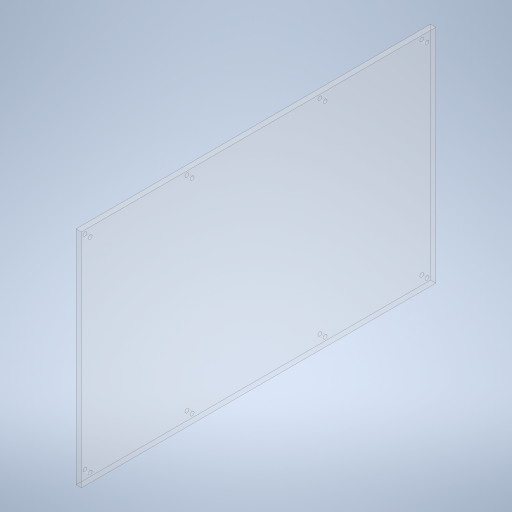
# Autodesk Inventor part: Perspex_plaat
Saved by Autodesk Inventor 2023 (Build 270158000, 158)
## iProperties
Created: 2022-09-12
Part Number: Perspex_plaat
Material: Polycarbonate, Clear
Document SubType Name: Modeling
Designer: VoorL
Density: 1.2 g/cm^3
Appearance: Polycarbonate - Clear
Author: VoorL
Autodesk Inventor part; units mm, degrees
ref_plane "YZ Plane" through (0, 0, 0) normal (1, 0, 0) x (0, 1, 0)
ref_plane "XZ Plane" through (0, 0, 0) normal (0, 1, 0) x (-1, 0, 0)
ref_plane "XY Plane" through (0, 0, 0) normal (0, 0, 1) x (1, 0, 0)
sketch "Sketch1" plane through (0, 0, 0) normal (1, 0, 0) x (0, 1, 0)
  line L0 (-125, 200) -> (125, 200)
  line L1 (125, 200) -> (125, -200)
  line L2 (125, -200) -> (-125, -200)
  line L3 (-125, -200) -> (-125, 200)
  line L4 (-125, 200) -> (125, -200) construction
  line L5 (125, 200) -> (-125, -200) construction
  point P0 (0, 0)
  dimension "d0" = 250
  dimension "d1" = 400
  constraints: 12 end point, 2 midpoint, 2 parallel, 1 horizontal, 1 perpendicular
  measures "d0" distance of L1.end L2.end
  measures "d1" distance of L0.end L1.end
extrude "Extrusion1" add sketch "Sketch1" along normal blind 6
sketch "Sketch2" plane through (6, 0, 0) normal (1, 0, 0) x (0, 0, -1)
  line L0 (-190, -115) -> (190, -115) construction
  line L1 (190, -115) -> (190, 115) construction
  line L2 (190, 115) -> (-190, 115) construction
  line L3 (-190, 115) -> (-190, -115) construction
  line L4 (-190, -115) -> (190, 115) construction
  line L5 (190, -115) -> (-190, 115) construction
  line L6 (-75, -115) -> (75, -115) construction
  line L7 (75, -115) -> (75, 115) construction
  line L8 (75, 115) -> (-75, 115) construction
  line L9 (-75, 115) -> (-75, -115) construction
  line L10 (-75, -115) -> (75, 115) construction
  line L11 (75, -115) -> (-75, 115) construction
  point P0 (0, 0)
  dimension "d4" = 380
  dimension "d5" = 230
  dimension "d6" = 150
  dimension "d7" = 230
  constraints: 24 end point, 4 midpoint, 4 parallel, 2 horizontal, 2 perpendicular
  measures "d4" distance of L2.end L1.end
  measures "d5" distance of L1.end L0.end
  measures "d6" distance of L8.end L7.end
  measures "d7" distance of L7.end L6.end
hole "Hole1" at (6, -115, 190) at (6, 115, -190) at (6, -115, -190) at (6, 115, 190) at (6, -115, 75) at (6, 115, -75) at (6, -115, -75) at (6, 115, 75) direction (-1, 0, 0) diameter 4.5 end through all
body "Solid1"
